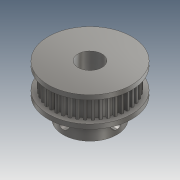
# Autodesk Inventor part: polia-gt2-40t-design1
Saved by Autodesk Inventor 2017 (Build 210142000, 142)
## iProperties
Created: 2018-05-19
Part Number: polia-gt2-40t-design1
Material: Stainless Steel
Document SubType Name: Modeling
Designer: Luiz Gustavo
Density: 8 g/cm^3
Appearance: Semi-Polished
Author: Luiz Gustavo
Autodesk Inventor part; units mm, degrees
ref_plane "YZ Plane" through (0, 0, 0) normal (1, 0, 0) x (0, 1, 0)
ref_plane "XZ Plane" through (0, 0, 0) normal (0, 1, 0) x (-1, 0, 0)
ref_plane "XY Plane" through (0, 0, 0) normal (0, 0, 1) x (1, 0, 0)
sketch "Sketch1" plane through (0, 0, 0) normal (0, 1, 0) x (-1, 0, 0)
  line L0 (0, -8.5) -> (0, 8.5) construction
  line L1 (0, 8.5) -> (-4, 8.5) construction
  line L2 (0, -8.5) -> (-4, -8.5) construction
  line L3 (-4, 8.5) -> (-4, -8.5)
  line L4 (-4, -8.5) -> (-9, -8.5)
  line L5 (-9, -8.5) -> (-9, -1.5)
  line L6 (-9, -1.5) -> (-14, -1.5)
  line L7 (-14, -1.5) -> (-14, 0)
  line L8 (-14, 0) -> (-12.5, 0)
  line L9 (-12.5, 0) -> (-12.5, 7)
  line L10 (-12.5, 7) -> (-14, 7)
  line L11 (-14, 7) -> (-14, 8.5)
  line L12 (-14, 8.5) -> (-4, 8.5)
  point P0 (0, 0)
  point P1 (0, 0)
  dimension "d0" = 17
  dimension "d1" = 8
  dimension "d4" = 10
  dimension "d5" = 1.5
  dimension "d6" = 1.5
  dimension "d8" = 25
  dimension "d9" = 28
  dimension "d11" = 18
  dimension "d12" = 7
  constraints: 26 end point, 6 perpendicular, 4 horizontal, 2 point on line, 2 vertical, 1 coincident, 1 midpoint
  measures "d0" distance of L0.start L0.end
  measures "d1" diameter of L3 L0
  measures "d4" distance between parallel lines of L6 L12
  measures "d5" distance of L10.end L11.end
  measures "d6" distance of L6.end L7.end
  measures "d8" diameter of L9 L0
  measures "d9" diameter of L11 L0
  measures "d11" diameter of L5 L0
  measures "d12" distance of L8.end L9.end
revolve "Revolution1" add sketch "Sketch1" angle 360 about axis through (0, 0, -8.5) along (0, 0, 1)
sketch "Sketch2" plane through (0, 0, 0) normal (1, 0, 0) x (0, 1, 0)
  circle A0 centre (0, -5) radius 2
  point P0 (0, 0)
  dimension "d13" = 4
  dimension "d18" = 5
  constraints: 1 centre point
  measures "d13" diameter of A0
  measures "d18" distance of A0.centre point (0, 0)
extrude "Extrusion1" cut sketch "Sketch2" along normal through all
sketch "Sketch3" plane through (0, 0, 0) normal (0, 1, 0) x (-1, 0, 0)
  circle A0 centre (0, -5) radius 2
  point P0 (0, 0)
  dimension "d16" = 4
  dimension "d17" = 5
  constraints: 1 centre point
  measures "d16" diameter of A0
  measures "d17" distance of A0.centre point (0, 0)
extrude "Extrusion2" cut sketch "Sketch3" against normal through all
sketch "Sketch4" plane through (0, 0, 0) normal (0, 0, 1) x (1, 0, 0)
  circle A0 centre (0, 0) radius 12.5 projected
  circle A1 centre (0, 0) radius 11.5 construction
  line L0 (0, -11.5) -> (0, -12.5) construction
  arc A2 (-0.5, -12.49) -> (0.5, -12.49) centre (0, 0) ccw
  line L1 (0.5, -12.49) -> (0.46, -11.4908)
  line L2 (-0.5, -12.49) -> (-0.46, -11.4908)
  arc A3 (-0.46, -11.4908) -> (0.46, -11.4908) centre (0, 0) ccw
  arc A4 (1.4124, -12.4199) -> (2.4007, -12.2673) centre (0, 0) ccw
  line L3 (2.4007, -12.2673) -> (2.2087, -11.2859)
  line L4 (1.4124, -12.4199) -> (1.2995, -11.4263)
  arc A5 (1.2995, -11.4263) -> (2.2087, -11.2859) centre (0, 0) ccw
  arc A6 (3.2918, -12.0588) -> (4.2452, -11.7571) centre (0, 0) ccw
  line L5 (4.2452, -11.7571) -> (3.9056, -10.8165)
  line L6 (3.2918, -12.0588) -> (3.0284, -11.0941)
  arc A7 (3.0284, -11.0941) -> (3.9056, -10.8165) centre (0, 0) ccw
  arc A8 (5.094, -11.415) -> (5.9901, -10.9712) centre (0, 0) ccw
  line L7 (5.9901, -10.9712) -> (5.5109, -10.0935)
  line L8 (5.094, -11.415) -> (4.6865, -10.5018)
  arc A9 (4.6865, -10.5018) -> (5.5109, -10.0935) centre (0, 0) ccw
  arc A10 (6.7768, -10.5036) -> (7.5947, -9.9283) centre (0, 0) ccw
  line L9 (7.5947, -9.9283) -> (6.9871, -9.134)
  line L10 (6.7768, -10.5036) -> (6.2346, -9.6633)
  arc A11 (6.2346, -9.6633) -> (6.9871, -9.134) centre (0, 0) ccw
  arc A12 (8.3007, -9.346) -> (9.0212, -8.6526) centre (0, 0) ccw
  line L11 (9.0212, -8.6526) -> (8.2995, -7.9604)
  line L12 (8.3007, -9.346) -> (7.6367, -8.5983)
  arc A13 (7.6367, -8.5983) -> (8.2995, -7.9604) centre (0, 0) ccw
  arc A14 (9.6301, -7.9694) -> (10.2363, -7.1741) centre (0, 0) ccw
  line L13 (10.2363, -7.1741) -> (9.4174, -6.6002)
  line L14 (9.6301, -7.9694) -> (8.8597, -7.3318)
  arc A15 (8.8597, -7.3318) -> (9.4174, -6.6002) centre (0, 0) ccw
  arc A16 (10.7338, -6.406) -> (11.2115, -5.5275) centre (0, 0) ccw
  line L15 (11.2115, -5.5275) -> (10.3146, -5.0853)
  line L16 (10.7338, -6.406) -> (9.8751, -5.8935)
  arc A17 (9.8751, -5.8935) -> (10.3146, -5.0853) centre (0, 0) ccw
  arc A18 (11.5858, -4.6924) -> (11.9238, -3.7513) centre (0, 0) ccw
  line L17 (11.9238, -3.7513) -> (10.9699, -3.4512)
  line L18 (11.5858, -4.6924) -> (10.659, -4.317)
  arc A19 (10.659, -4.317) -> (10.9699, -3.4512) centre (0, 0) ccw
  arc A20 (12.1663, -2.8688) -> (12.3567, -1.8871) centre (0, 0) ccw
  line L19 (12.3567, -1.8871) -> (11.3682, -1.7362)
  line L20 (12.1663, -2.8688) -> (11.193, -2.6393)
  arc A21 (11.193, -2.6393) -> (11.3682, -1.7362) centre (0, 0) ccw
  arc A22 (12.4617, -0.978) -> (12.5, 0.0212) centre (0, 0) ccw
  line L21 (12.5, 0.0212) -> (11.5, 0.0195)
  line L22 (12.4617, -0.978) -> (11.4647, -0.8998)
  arc A23 (11.4647, -0.8998) -> (11.5, 0.0195) centre (0, 0) ccw
  arc A24 (12.4649, 0.9357) -> (12.3502, 1.9291) centre (0, 0) ccw
  line L23 (12.3502, 1.9291) -> (11.3622, 1.7748)
  line L24 (12.4649, 0.9357) -> (11.4677, 0.8608)
  arc A25 (11.4677, 0.8608) -> (11.3622, 1.7748) centre (0, 0) ccw
  arc A26 (12.176, 2.8275) -> (11.911, 3.7917) centre (0, 0) ccw
  line L25 (11.911, 3.7917) -> (10.9581, 3.4884)
  line L26 (12.176, 2.8275) -> (11.2019, 2.6013)
  arc A27 (11.2019, 2.6013) -> (10.9581, 3.4884) centre (0, 0) ccw
  arc A28 (11.6017, 4.653) -> (11.1926, 5.5655) centre (0, 0) ccw
  line L27 (11.1926, 5.5655) -> (10.2972, 5.1203)
  line L28 (11.6017, 4.653) -> (10.6736, 4.2808)
  arc A29 (10.6736, 4.2808) -> (10.2972, 5.1203) centre (0, 0) ccw
  arc A30 (10.7555, 6.3695) -> (10.2119, 7.2088) centre (0, 0) ccw
  line L29 (10.2119, 7.2088) -> (9.3949, 6.6321)
  line L30 (10.7555, 6.3695) -> (9.895, 5.8599)
  arc A31 (9.895, 5.8599) -> (9.3949, 6.6321) centre (0, 0) ccw
  arc A32 (9.6571, 7.9366) -> (8.9918, 8.6832) centre (0, 0) ccw
  line L31 (8.9918, 8.6832) -> (8.2724, 7.9885)
  line L32 (9.6571, 7.9366) -> (8.8845, 7.3017)
  arc A33 (8.8845, 7.3017) -> (8.2724, 7.9885) centre (0, 0) ccw
  arc A34 (8.3324, 9.3178) -> (7.5609, 9.954) centre (0, 0) ccw
  line L33 (7.5609, 9.954) -> (6.956, 9.1577)
  line L34 (8.3324, 9.3178) -> (7.6658, 8.5724)
  arc A35 (7.6658, 8.5724) -> (6.956, 9.1577) centre (0, 0) ccw
  arc A36 (6.8124, 10.4805) -> (5.9528, 10.9915) centre (0, 0) ccw
  line L35 (5.9528, 10.9915) -> (5.4766, 10.1122)
  line L36 (6.8124, 10.4805) -> (6.2674, 9.6421)
  arc A37 (6.2674, 9.6421) -> (5.4766, 10.1122) centre (0, 0) ccw
  arc A38 (5.1327, 11.3976) -> (4.2052, 11.7714) centre (0, 0) ccw
  line L37 (4.2052, 11.7714) -> (3.8688, 10.8297)
  line L38 (5.1327, 11.3976) -> (4.7221, 10.4858)
  arc A39 (4.7221, 10.4858) -> (3.8688, 10.8297) centre (0, 0) ccw
  arc A40 (3.3327, 12.0475) -> (2.359, 12.2754) centre (0, 0) ccw
  line L39 (2.359, 12.2754) -> (2.1703, 11.2933)
  line L40 (3.3327, 12.0475) -> (3.0661, 11.0837)
  arc A41 (3.0661, 11.0837) -> (2.1703, 11.2933) centre (0, 0) ccw
  arc A42 (1.4546, 12.4151) -> (0.4576, 12.4916) centre (0, 0) ccw
  line L41 (0.4576, 12.4916) -> (0.421, 11.4923)
  line L42 (1.4546, 12.4151) -> (1.3383, 11.4219)
  arc A43 (1.3383, 11.4219) -> (0.421, 11.4923) centre (0, 0) ccw
  arc A44 (-0.4576, 12.4916) -> (-1.4546, 12.4151) centre (0, 0) ccw
  line L43 (-1.4546, 12.4151) -> (-1.3383, 11.4219)
  line L44 (-0.4576, 12.4916) -> (-0.421, 11.4923)
  arc A45 (-0.421, 11.4923) -> (-1.3383, 11.4219) centre (0, 0) ccw
  arc A46 (-2.359, 12.2754) -> (-3.3327, 12.0475) centre (0, 0) ccw
  line L45 (-3.3327, 12.0475) -> (-3.0661, 11.0837)
  line L46 (-2.359, 12.2754) -> (-2.1703, 11.2933)
  arc A47 (-2.1703, 11.2933) -> (-3.0661, 11.0837) centre (0, 0) ccw
  arc A48 (-4.2052, 11.7714) -> (-5.1327, 11.3976) centre (0, 0) ccw
  line L47 (-5.1327, 11.3976) -> (-4.7221, 10.4858)
  line L48 (-4.2052, 11.7714) -> (-3.8688, 10.8297)
  arc A49 (-3.8688, 10.8297) -> (-4.7221, 10.4858) centre (0, 0) ccw
  arc A50 (-5.9528, 10.9915) -> (-6.8124, 10.4805) centre (0, 0) ccw
  line L49 (-6.8124, 10.4805) -> (-6.2674, 9.6421)
  line L50 (-5.9528, 10.9915) -> (-5.4766, 10.1122)
  arc A51 (-5.4766, 10.1122) -> (-6.2674, 9.6421) centre (0, 0) ccw
  arc A52 (-7.5609, 9.954) -> (-8.3324, 9.3178) centre (0, 0) ccw
  line L51 (-8.3324, 9.3178) -> (-7.6658, 8.5724)
  line L52 (-7.5609, 9.954) -> (-6.956, 9.1577)
  arc A53 (-6.956, 9.1577) -> (-7.6658, 8.5724) centre (0, 0) ccw
  arc A54 (-8.9918, 8.6832) -> (-9.6571, 7.9366) centre (0, 0) ccw
  line L53 (-9.6571, 7.9366) -> (-8.8845, 7.3017)
  line L54 (-8.9918, 8.6832) -> (-8.2724, 7.9885)
  arc A55 (-8.2724, 7.9885) -> (-8.8845, 7.3017) centre (0, 0) ccw
  arc A56 (-10.2119, 7.2088) -> (-10.7555, 6.3695) centre (0, 0) ccw
  line L55 (-10.7555, 6.3695) -> (-9.895, 5.8599)
  line L56 (-10.2119, 7.2088) -> (-9.3949, 6.6321)
  arc A57 (-9.3949, 6.6321) -> (-9.895, 5.8599) centre (0, 0) ccw
  arc A58 (-11.1926, 5.5655) -> (-11.6017, 4.653) centre (0, 0) ccw
  line L57 (-11.6017, 4.653) -> (-10.6736, 4.2808)
  line L58 (-11.1926, 5.5655) -> (-10.2972, 5.1203)
  arc A59 (-10.2972, 5.1203) -> (-10.6736, 4.2808) centre (0, 0) ccw
  arc A60 (-11.911, 3.7917) -> (-12.176, 2.8275) centre (0, 0) ccw
  line L59 (-12.176, 2.8275) -> (-11.2019, 2.6013)
  line L60 (-11.911, 3.7917) -> (-10.9581, 3.4884)
  arc A61 (-10.9581, 3.4884) -> (-11.2019, 2.6013) centre (0, 0) ccw
  arc A62 (-12.3502, 1.9291) -> (-12.4649, 0.9357) centre (0, 0) ccw
  line L61 (-12.4649, 0.9357) -> (-11.4677, 0.8608)
  line L62 (-12.3502, 1.9291) -> (-11.3622, 1.7748)
  arc A63 (-11.3622, 1.7748) -> (-11.4677, 0.8608) centre (0, 0) ccw
  arc A64 (-12.5, 0.0212) -> (-12.4617, -0.978) centre (0, 0) ccw
  line L63 (-12.4617, -0.978) -> (-11.4647, -0.8998)
  line L64 (-12.5, 0.0212) -> (-11.5, 0.0195)
  arc A65 (-11.5, 0.0195) -> (-11.4647, -0.8998) centre (0, 0) ccw
  arc A66 (-12.3567, -1.8871) -> (-12.1663, -2.8688) centre (0, 0) ccw
  line L65 (-12.1663, -2.8688) -> (-11.193, -2.6393)
  line L66 (-12.3567, -1.8871) -> (-11.3682, -1.7362)
  arc A67 (-11.3682, -1.7362) -> (-11.193, -2.6393) centre (0, 0) ccw
  arc A68 (-11.9238, -3.7513) -> (-11.5858, -4.6924) centre (0, 0) ccw
  line L67 (-11.5858, -4.6924) -> (-10.659, -4.317)
  line L68 (-11.9238, -3.7513) -> (-10.9699, -3.4512)
  arc A69 (-10.9699, -3.4512) -> (-10.659, -4.317) centre (0, 0) ccw
  arc A70 (-11.2115, -5.5275) -> (-10.7338, -6.406) centre (0, 0) ccw
  line L69 (-10.7338, -6.406) -> (-9.8751, -5.8935)
  line L70 (-11.2115, -5.5275) -> (-10.3146, -5.0853)
  arc A71 (-10.3146, -5.0853) -> (-9.8751, -5.8935) centre (0, 0) ccw
  arc A72 (-10.2363, -7.1741) -> (-9.6301, -7.9694) centre (0, 0) ccw
  line L71 (-9.6301, -7.9694) -> (-8.8597, -7.3318)
  line L72 (-10.2363, -7.1741) -> (-9.4174, -6.6002)
  arc A73 (-9.4174, -6.6002) -> (-8.8597, -7.3318) centre (0, 0) ccw
  arc A74 (-9.0212, -8.6526) -> (-8.3007, -9.346) centre (0, 0) ccw
  line L73 (-8.3007, -9.346) -> (-7.6367, -8.5983)
  line L74 (-9.0212, -8.6526) -> (-8.2995, -7.9604)
  arc A75 (-8.2995, -7.9604) -> (-7.6367, -8.5983) centre (0, 0) ccw
  arc A76 (-7.5947, -9.9283) -> (-6.7768, -10.5036) centre (0, 0) ccw
  line L75 (-6.7768, -10.5036) -> (-6.2346, -9.6633)
  line L76 (-7.5947, -9.9283) -> (-6.9871, -9.134)
  arc A77 (-6.9871, -9.134) -> (-6.2346, -9.6633) centre (0, 0) ccw
  arc A78 (-5.9901, -10.9712) -> (-5.094, -11.415) centre (0, 0) ccw
  line L77 (-5.094, -11.415) -> (-4.6865, -10.5018)
  line L78 (-5.9901, -10.9712) -> (-5.5109, -10.0935)
  arc A79 (-5.5109, -10.0935) -> (-4.6865, -10.5018) centre (0, 0) ccw
  arc A80 (-4.2452, -11.7571) -> (-3.2918, -12.0588) centre (0, 0) ccw
  line L79 (-3.2918, -12.0588) -> (-3.0284, -11.0941)
  line L80 (-4.2452, -11.7571) -> (-3.9056, -10.8165)
  arc A81 (-3.9056, -10.8165) -> (-3.0284, -11.0941) centre (0, 0) ccw
  arc A82 (-2.4007, -12.2673) -> (-1.4124, -12.4199) centre (0, 0) ccw
  line L81 (-1.4124, -12.4199) -> (-1.2995, -11.4263)
  line L82 (-2.4007, -12.2673) -> (-2.2087, -11.2859)
  arc A83 (-2.2087, -11.2859) -> (-1.2995, -11.4263) centre (0, 0) ccw
  point P0 (0, 0)
  point P1 (1.7555, -11.3652)
  point P2 (1.9081, -12.3535)
  point P3 (3.4698, -10.9641)
  point P4 (3.7715, -11.9175)
  point P5 (5.1028, -10.3059)
  point P6 (5.5465, -11.2021)
  point P7 (6.6162, -9.4062)
  point P8 (7.1915, -10.2241)
  point P9 (7.9745, -8.286)
  point P10 (8.6679, -9.0065)
  point P11 (9.1459, -6.9716)
  point P12 (9.9412, -7.5778)
  point P13 (10.1029, -5.4938)
  point P14 (10.9814, -5.9715)
  point P15 (10.8231, -3.8872)
  point P16 (11.7643, -4.2252)
  point P17 (11.2896, -2.1895)
  point P18 (12.2714, -2.3799)
  point P19 (11.4916, -0.4405)
  point P20 (12.4908, -0.4788)
  point P21 (11.4241, 1.3189)
  point P22 (12.4175, 1.4335)
  point P23 (11.0889, 3.0473)
  point P24 (12.0532, 3.3123)
  point P25 (10.4938, 4.7043)
  point P26 (11.4063, 5.1134)
  point P27 (9.6527, 6.251)
  point P28 (10.4921, 6.7946)
  point P29 (8.5854, 7.6512)
  point P30 (9.3319, 8.3166)
  point P31 (7.3168, 8.8721)
  point P32 (7.953, 9.6436)
  point P33 (5.8767, 9.8851)
  point P34 (6.3877, 10.7446)
  point P35 (4.2989, 10.6663)
  point P36 (4.6727, 11.5938)
  point P37 (2.6203, 11.1975)
  point P38 (2.8482, 12.1712)
  point P39 (0.8803, 11.4663)
  point P40 (0.9569, 12.4633)
  point P41 (-0.8803, 11.4663)
  point P42 (-0.9569, 12.4633)
  point P43 (-2.6203, 11.1975)
  point P44 (-2.8482, 12.1712)
  point P45 (-4.2989, 10.6663)
  point P46 (-4.6727, 11.5938)
  point P47 (-5.8767, 9.8851)
  point P48 (-6.3877, 10.7446)
  point P49 (-7.3168, 8.8721)
  point P50 (-7.953, 9.6436)
  point P51 (-8.5854, 7.6512)
  point P52 (-9.3319, 8.3166)
  point P53 (-9.6527, 6.251)
  point P54 (-10.4921, 6.7946)
  point P55 (-10.4938, 4.7043)
  point P56 (-11.4063, 5.1134)
  point P57 (-11.0889, 3.0473)
  point P58 (-12.0532, 3.3123)
  point P59 (-11.4241, 1.3189)
  point P60 (-12.4175, 1.4335)
  point P61 (-11.4916, -0.4405)
  point P62 (-12.4908, -0.4788)
  point P63 (-11.2896, -2.1895)
  point P64 (-12.2714, -2.3799)
  point P65 (-10.8231, -3.8872)
  point P66 (-11.7643, -4.2252)
  point P67 (-10.1029, -5.4938)
  point P68 (-10.9814, -5.9715)
  point P69 (-9.1459, -6.9716)
  point P70 (-9.9412, -7.5778)
  point P71 (-7.9745, -8.286)
  point P72 (-8.6679, -9.0065)
  point P73 (-6.6162, -9.4062)
  point P74 (-7.1915, -10.2241)
  point P75 (-5.1028, -10.3059)
  point P76 (-5.5465, -11.2021)
  point P77 (-3.4698, -10.9641)
  point P78 (-3.7715, -11.9175)
  point P79 (-1.7555, -11.3652)
  point P80 (-1.9081, -12.3535)
  dimension "d21" = 1
  dimension "d22" = 1
  dimension "d25" = 360
  constraints: 169 point on circle, 166 end point, 83 centre point, 43 coincident, 1 concentric, 1 line through centre, 1 symmetric about line, 1 vertical, 494 other
  measures "d21" distance of L1.start L2.start
  measures "d22" radial gap between concentric circles of A1 A0
extrude "Extrusion3" cut sketch "Sketch4" along normal up to surface (7 mm away) contours A0 L22 A23 L21 | L24 A25 L23 A0 | A0 L20 A21 L19 | L26 A27 L25 A0 | A0 L18 A19 L17 | L28 A29 L27 A0 | A0 L16 A17 L15 | L30 A31 L29 A0 | A0 L14 A15 L13 | L32 A33 L31 A0 | A0 L12 A13 L11 | L34 A35 L33 A0 | A0 L10 A11 L9 | L36 A37 L35 A0 | A0 L8 A9 L7 | L38 A39 L37 A0 | A0 L6 A7 L5 | L40 A41 L39 A0 | A0 L4 A5 L3 | L42 A43 L41 A0 | A0 L2 A3 L1 | L44 A45 L43 A0 | A0 L82 A83 L81 | L46 A47 L45 A0 | A0 L80 A81 L79 | L48 A49 L47 A0 | A0 L78 A79 L77 | L50 A51 L49 A0 | A0 L76 A77 L75 | L52 A53 L51 A0 | A0 L74 A75 L73 | L54 A55 L53 A0 | A0 L72 A73 L71 | L56 A57 L55 A0 | A0 L70 A71 L69 | L58 A59 L57 A0 | A0 L68 A69 L67 | L60 A61 L59 A0 | A0 L66 A67 L65 | L62 A63 L61 A0 | A0 L64 A65 L63
chamfer "Chamfer1" distance 0.2 angle 45 82 edges at (6.7768, -10.5036, 3.5) (5.9901, -10.9712, 3.5) (5.094, -11.415, 3.5) (4.2452, -11.7571, 3.5) (3.2918, -12.0588, 3.5) (2.4007, -12.2673, 3.5) (1.4124, -12.4199, 3.5) (0.5, -12.49, 3.5) (-0.5, -12.49, 3.5) (-1.4124, -12.4199, 3.5) (-2.4007, -12.2673, 3.5) (-3.2918, -12.0588, 3.5) (-4.2452, -11.7571, 3.5) (-5.094, -11.415, 3.5) (-5.9901, -10.9712, 3.5) (-6.7768, -10.5036, 3.5) (-7.5947, -9.9283, 3.5) (-8.3007, -9.346, 3.5) (-9.0212, -8.6526, 3.5) (-9.6301, -7.9694, 3.5) (-10.2363, -7.1741, 3.5) (-10.7338, -6.406, 3.5) (-11.5858, -4.6924, 3.5) (-11.2115, -5.5275, 3.5) (-11.9238, -3.7513, 3.5) (-12.1663, -2.8688, 3.5) (-12.3567, -1.8871, 3.5) (-12.4617, -0.978, 3.5) (-12.5, 0.0212, 3.5) (-12.4649, 0.9357, 3.5) (-12.3502, 1.9291, 3.5) (-12.176, 2.8275, 3.5) (-11.911, 3.7917, 3.5) (-11.6017, 4.653, 3.5) (-11.1926, 5.5655, 3.5) (-10.7555, 6.3695, 3.5) (-10.2119, 7.2088, 3.5) (-9.6571, 7.9366, 3.5) (-8.9918, 8.6832, 3.5) (-8.3324, 9.3178, 3.5) (-7.5609, 9.954, 3.5) (-6.8124, 10.4805, 3.5) (-5.9528, 10.9915, 3.5) (-5.1327, 11.3976, 3.5) (-4.2052, 11.7714, 3.5) (-3.3327, 12.0475, 3.5) (-2.359, 12.2754, 3.5) (-1.4546, 12.4151, 3.5) (-0.4576, 12.4916, 3.5) (0.4576, 12.4916, 3.5) (1.4546, 12.4151, 3.5) (2.359, 12.2754, 3.5) (3.3327, 12.0475, 3.5) (4.2052, 11.7714, 3.5) (5.1327, 11.3976, 3.5) (5.9528, 10.9915, 3.5) (6.8124, 10.4805, 3.5) (7.5609, 9.954, 3.5) (8.3324, 9.3178, 3.5) (8.9918, 8.6832, 3.5) (9.6571, 7.9366, 3.5) (10.2119, 7.2088, 3.5) (10.7555, 6.3695, 3.5) (11.1926, 5.5655, 3.5) (11.6017, 4.653, 3.5) (11.911, 3.7917, 3.5) (12.176, 2.8275, 3.5) (12.3502, 1.9291, 3.5) (12.4649, 0.9357, 3.5) (12.5, 0.0212, 3.5) (12.4617, -0.978, 3.5) (12.3567, -1.8871, 3.5) (12.1663, -2.8688, 3.5) (11.9238, -3.7513, 3.5) (11.5858, -4.6924, 3.5) (11.2115, -5.5275, 3.5) (10.7338, -6.406, 3.5) (10.2363, -7.1741, 3.5) (9.6301, -7.9694, 3.5) (9.0212, -8.6526, 3.5) (8.3007, -9.346, 3.5) (7.5947, -9.9283, 3.5)
equation "\"d5\" = d6"
body "Solid1"
